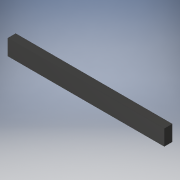
# Autodesk Inventor part: PiGPIOBase
Saved by Autodesk Inventor 2018 (Build 220112000, 112)
## iProperties
Created: 2018-01-13
Part Number: PiGPIOBase
Material: ABS Plastic
Document SubType Name: Modeling
Designer: Kyle-HP
Density: 1.06 g/cm^3
Appearance: Smooth - Black
Author: Kyle-HP
Autodesk Inventor part; units mm, degrees
ref_plane "YZ Plane" through (0, 0, 0) normal (1, 0, 0) x (0, 1, 0)
ref_plane "XZ Plane" through (0, 0, 0) normal (0, 1, 0) x (-1, 0, 0)
ref_plane "XY Plane" through (0, 0, 0) normal (0, 0, 1) x (1, 0, 0)
sketch "Sketch1" plane through (0, 0, 0) normal (0, 0, 1) x (1, 0, 0)
  line L0 (0, 0) -> (50.8, 0)
  line L1 (50.8, 0) -> (50.8, -5.08)
  line L2 (50.8, -5.08) -> (0, -5.08)
  line L3 (0, -5.08) -> (0, 0)
  dimension "d0" = 50.8
  dimension "d1" = 5.08
  constraints: 8 end point, 2 parallel, 1 horizontal, 1 perpendicular
  measures "d0" distance of L0.start L0.end
  measures "d1" distance of L2.end L0.start
extrude "Extrusion1" add sketch "Sketch1" along normal blind 2.54
body "Solid1"
